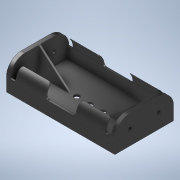
# Autodesk Inventor part: Main body
Saved by Autodesk Inventor 2020 (Build 240168000, 168)
## iProperties
Created: 2021-12-31
Part Number: Main body
Material: ABS Plastic
Document SubType Name: Modeling
Designer: robur
Density: 1.06 g/cm^3
Appearance: Asphalt 2
Author: robur
Autodesk Inventor part; units mm, degrees
ref_plane "YZ Plane" through (0, 0, 0) normal (1, 0, 0) x (0, 1, 0)
sketch "Sketch2" plane through (0, 0, 0) normal (0, 1, 0) x (-1, 0, 0)
  line L0 (28.8, 15.6) -> (-28.8, 15.6)
  line L1 (-28.8, 15.6) -> (-28.8, -15.6)
  line L2 (-28.8, -15.6) -> (28.8, -15.6)
  line L3 (28.8, -15.6) -> (28.8, 15.6)
  line L4 (28.8, 15.6) -> (-28.8, -15.6) construction
  line L5 (-28.8, 15.6) -> (28.8, -15.6) construction
  circle A0 centre (7, 0) radius 1.4
  circle A1 centre (0, 0) radius 1.4
  circle A2 centre (-7, 0) radius 1.4
  dimension "d0" = 57.6
  dimension "d1" = 31.2
  dimension "d2" = 2.8
  dimension "d3" = 21.8
  dimension "d4" = 2.8
  dimension "d5" = 2.8
  dimension "d6" = 7
  dimension "d7" = 7
  constraints: 12 end point, 3 centre point, 2 midpoint, 2 parallel, 1 coincident, 1 horizontal, 1 perpendicular
  measures "d0" distance of L2.end L1.end
  measures "d1" distance of L1.end L0.end
  measures "d2" diameter of A0
  measures "d3" distance from line of A0.centre L3
  measures "d4" diameter of A1
  measures "d5" diameter of A2
  measures "d6" distance of A2.centre point (0, 0)
  measures "d7" distance of point (0, 0) A0.centre
extrude "Extrusion1" add sketch "Sketch2" along normal blind 15
fillet "Fillet1" radius 8 2 edges at (0, 15, 15.6) (0, 15, -15.6)
ref_plane "Work Plane1" through (26.8, 0, 15.6) normal (1, 0, 0) x (0, 0, -1)
sketch "Sketch3" plane through (26.8, 0, 15.6) normal (1, 0, 0) x (0, 0, -1)
  arc A0 (8, 15) -> (0, 7) centre (8, 7) ccw
  arc A1 (8, 15) -> (0, 7) centre (8, 7) ccw projected
  arc A2 (8, 14) -> (1, 7) centre (8, 7) ccw
  arc A3 (31.2, 7) -> (23.2, 15) centre (23.2, 7) ccw projected
  arc A4 (30.2, 7) -> (23.2, 14) centre (23.2, 7) ccw
  line L0 (1, 7) -> (1, 1)
  line L1 (31.2, 0) -> (0, 0) projected
  line L2 (1, 1) -> (30.2, 1)
  line L3 (31.2, 0) -> (31.2, 7) projected
  line L4 (30.2, 1) -> (30.2, 7)
  line L5 (23.2, 15) -> (8, 15)
  line L6 (23.2, 14) -> (8, 14)
  point P0 (15.6, 0)
  dimension "d12" = 7
  dimension "d13" = 7
  dimension "d14" = 6
  dimension "d15" = 29.2
  constraints: 10 end point, 6 point on circle, 3 centre point, 3 coincident, 2 perpendicular, 1 horizontal, 1 parallel, 1 tangent
  measures "d12" radius of A2
  measures "d13" radius of A4
  measures "d14" distance of L0.start L0.end
  measures "d15" distance of L0.end L2.end
extrude "Extrusion2" cut sketch "Sketch3" against normal blind 53.6
sketch "Sketch4" plane through (0, 15, 0) normal (0, 1, 0) x (1, 0, 0)
  line L0 (26.8, -14.6) -> (26.8, 14.6) projected
  line L1 (-26.8, -12.5) -> (26.8, -12.5)
  line L2 (26.8, -12.5) -> (26.8, 12.5)
  line L3 (26.8, 12.5) -> (-26.8, 12.5)
  line L4 (-26.8, 12.5) -> (-26.8, -12.5)
  line L5 (-26.8, -12.5) -> (26.8, 12.5) construction
  line L6 (26.8, -12.5) -> (-26.8, 12.5) construction
  point P0 (0, 0)
  dimension "d51" = 25
  constraints: 12 end point, 2 midpoint, 2 parallel, 1 horizontal, 1 perpendicular, 1 point on line
  measures "d51" distance of L3.end L1.start
extrude "Extrusion3" cut sketch "Sketch4" against normal blind 3
ref_plane "Work Plane2" through (28.8, 0, -15.6) normal (0, 0, -1) x (-1, 0, 0)
sketch "Sketch8" plane through (-26.8, 0, 15.6) normal (1, 0, 0) x (0, 0, -1)
  line L0 (3.1, 13.3238) -> (3.1, 12) projected
  arc A0 (3.1, 13.0156) -> (1, 7) centre (6.8512, 8.3318) ccw
  line L1 (8, 15) -> (23.2, 15) projected
  line L2 (15.6, 15) -> (15.6, 0.9201)
  arc A1 (30.2, 7) -> (28.1, 13.0156) centre (24.3488, 8.3318) ccw
  line L3 (28.1, 13.0156) -> (3.1, 13.0156)
  arc A2 (30.2, 7) -> (28.099, 12) centre (23.2, 7) ccw projected
  line L4 (1, 7) -> (30.2, 7)
  point P0 (15.6, 0)
  constraints: 6 end point, 4 point on circle, 3 symmetric about line, 2 centre point, 1 horizontal, 1 midpoint, 1 parallel, 1 point on line, 1 vertical, 1 other
extrude "Extrusion6" cut sketch "Sketch8" along normal blind 53.6
sketch "Sketch9" plane through (28.8, 0, -15.6) normal (0, 0, -1) x (-1, 0, 0)
  line L0 (2, 13.3238) -> (5, 13.3238)
  line L1 (5, 11.8238) -> (5, 8.2996)
  line L2 (3.5, 6.7996) -> (2, 6.7996)
  line L3 (2, 6.7996) -> (2, 13.3238)
  arc A0 (3.5, 6.7996) -> (5, 8.2996) centre (3.5, 8.2996) ccw
  arc A1 (6.5, 13.3238) -> (5, 11.8238) centre (6.5, 11.8238) ccw
  line L4 (5, 13.3238) -> (6.5, 13.3238)
  line L5 (28.8, 0) -> (28.8, 13.3238)
  line L6 (55.6, 13.3238) -> (52.6, 13.3238)
  line L7 (52.6, 11.8238) -> (52.6, 8.2996)
  line L8 (54.1, 6.7996) -> (55.6, 6.7996)
  line L9 (55.6, 6.7996) -> (55.6, 13.3238)
  arc A2 (52.6, 8.2996) -> (54.1, 6.7996) centre (54.1, 8.2996) ccw
  arc A3 (52.6, 11.8238) -> (51.1, 13.3238) centre (51.1, 11.8238) ccw
  line L10 (52.6, 13.3238) -> (51.1, 13.3238)
  line L11 (55.6, 13.3238) -> (2, 13.3238) projected
  line L12 (2, 7) -> (55.6, 7) projected
  line L13 (20.85, 13.3238) -> (36.75, 13.3238)
  line L14 (36.75, 11.8238) -> (36.75, 8.5)
  line L15 (35.25, 7) -> (22.35, 7)
  line L16 (20.85, 8.5) -> (20.85, 11.8238)
  arc A4 (20.85, 8.5) -> (22.35, 7) centre (22.35, 8.5) ccw
  arc A5 (35.25, 7) -> (36.75, 8.5) centre (35.25, 8.5) ccw
  arc A6 (38.25, 13.3238) -> (36.75, 11.8238) centre (38.25, 11.8238) ccw
  arc A7 (20.85, 11.8238) -> (19.35, 13.3238) centre (19.35, 11.8238) ccw
  line L17 (20.85, 13.3238) -> (19.35, 13.3238)
  line L18 (36.75, 13.3238) -> (38.25, 13.3238)
  point P0 (53.3509, 7)
  point P1 (4.2491, 7)
  dimension "d55" = 3
  dimension "d57" = 1.5
  dimension "d58" = 1.5
  dimension "d59" = 3
  dimension "d60" = 1.5
  dimension "d63" = 15.85
  dimension "d64" = 3
  dimension "d65" = 1.5
  dimension "d66" = 1.5
  dimension "d67" = 3
  dimension "d68" = 1.5
  dimension "d69" = 1.5
  dimension "d70" = 3
  dimension "d71" = 1.5
  dimension "d72" = 1.5
  dimension "d73" = 3
  dimension "d74" = 1.5
  dimension "d75" = 1.5
  constraints: 34 end point, 16 point on circle, 9 symmetric about line, 8 centre point, 4 parallel, 2 horizontal, 2 perpendicular, 6 other
  measures "d55" diameter of A0
  measures "d57" distance from line of L1 A0.centre
  measures "d58" distance from line of L2 A0.centre
  measures "d59" diameter of A1
  measures "d60" distance from line of L1 A1.centre
  measures "d63" distance between parallel lines of L7 L14
  measures "d64" diameter of A4
  measures "d65" distance from line of L12 A4.centre
  measures "d66" distance from line of L16 A4.centre
  measures "d67" diameter of A5
  measures "d68" distance from line of L14 A5.centre
  measures "d69" distance from line of L12 A5.centre
  measures "d70" diameter of A6
  measures "d71" distance from line of L14 A6.centre
  measures "d72" distance from line of L13 A6.centre
  measures "d73" diameter of A7
  measures "d74" distance from line of L16 A7.centre
  measures "d75" distance from line of L13 A7.centre
extrude "Extrusion7" cut sketch "Sketch9" against normal blind 53.8 contours L0 L4 A1 L1 A0 L12 L3 | L11 L5 L12 A4 L16 A7 | L5 L11 A6 L14 A5 L12 | A2 L7 A3 L10 L6 L9 L12
sketch "Sketch10" plane through (26.8, 1, 14.6) normal (0, 1, 0) x (1, 0, 0)
  line L0 (0, 0) -> (0, 29.2) projected
  line L1 (0, 14.1) -> (0, 15.1)
  line L2 (-53.6, 15.1) -> (-53.6, 14.1)
  circle A0 centre (-26.8, 14.6) radius 1.4 projected
  line L3 (-53.6, 14.1) -> (0, 15.1) construction
  line L4 (0, 14.1) -> (-53.6, 15.1) construction
  line L5 (-37.3, 14.1) -> (-37.3, 15.1)
  circle A1 centre (-33.8, 14.6) radius 1.4 projected
  line L6 (-16.3, 15.1) -> (-16.3, 14.1)
  circle A2 centre (-19.8, 14.6) radius 1.4 projected
  line L7 (-53.6, 14.1) -> (-37.3, 14.1)
  line L8 (-16.3, 14.1) -> (0, 14.1)
  line L9 (0, 15.1) -> (-16.3, 15.1)
  line L10 (-37.3, 15.1) -> (-53.6, 15.1)
  dimension "d78" = 1
  dimension "d79" = 3.5
  dimension "d80" = 3.5
  constraints: 20 end point, 6 perpendicular, 5 parallel, 2 horizontal, 2 midpoint, 1 point on line
  measures "d78" distance of L1.end L1.start
  measures "d79" distance from line of L5 A1.centre
  measures "d80" distance from line of L6 A2.centre
extrude "Extrusion8" add sketch "Sketch10" along normal blind 14 contours L8 L6 L9 L0 | L10 L5 L7 L2
sketch "Sketch11" plane through (-26.8, 1, 0.5) normal (0, 0, 1) x (1, 0, 0)
  line L0 (16.3, 14) -> (0, 14) projected
  line L1 (16.3, 0) -> (0, 0) projected
  line L2 (0, 14) -> (16.3, 0)
  line L3 (16.3, 0) -> (16.3, 14)
  line L4 (20.35, 6) -> (2.2491, 6) projected
  line L5 (0, 14) -> (16.3, 14) projected
  line L6 (16.3, 14) -> (0, 14)
  point P0 (26.8, -1)
  constraints: 6 end point, 2 perpendicular
extrude "Extrusion9" cut sketch "Sketch11" against normal blind 1
sketch "Sketch12" plane through (10.5, 1, 0.5) normal (0, 0, 1) x (1, 0, 0)
  line L0 (16.3, 0) -> (0, 0) projected
  line L1 (16.3, 14) -> (0, 0)
  line L2 (0, 14) -> (16.3, 14) projected
  line L3 (0, 0) -> (0, 14)
  line L4 (16.3, 0) -> (16.3, 14) projected
  line L5 (0, 14) -> (16.3, 14)
  point P0 (-10.5, -1)
  constraints: 6 end point, 2 perpendicular
extrude "Extrusion10" cut sketch "Sketch12" against normal blind 1 contours L3 L2 L1
sketch "Sketch13" plane through (28.8, 0, 15.6) normal (1, 0, 0) x (0, 0, -1)
  circle A0 centre (8, 7.8) radius 0.9
  line L0 (8, 15) -> (23.2, 15) projected
  line L1 (0, 0) -> (0, 7) projected
  line L2 (15.6, 0) -> (15.6, 15)
  line L3 (31.2, 0) -> (31.2, 7) projected
  circle A1 centre (23.2, 7.8) radius 0.9
  dimension "d87" = 1.8
  dimension "d88" = 7.2
  dimension "d89" = 8
  dimension "d90" = 15.6
  dimension "d91" = 15.6
  constraints: 2 centre point, 2 end point, 1 midpoint, 1 symmetric about line, 1 other
  measures "d87" diameter of A0
  measures "d88" distance from line of L0 A0.centre
  measures "d89" distance from line of L1 A0.centre
  measures "d90" distance between parallel lines of L2 L1
  measures "d91" distance between parallel lines of L3 L2
extrude "Extrusion11" cut sketch "Sketch13" against normal blind 2
sketch "Sketch14" plane through (-26.8, 0, 15.6) normal (1, 0, 0) x (0, 0, -1)
  circle A0 centre (8, 7.8) radius 0.9 projected
  circle A1 centre (8, 7.8) radius 0.9
  circle A2 centre (23.2, 7.8) radius 0.9 projected
  circle A3 centre (23.2, 7.8) radius 0.9
  point P0 (15.6, 0)
  constraints: 2 centre point, 2 coincident
extrude "Extrusion12" cut sketch "Sketch14" against normal blind 2
body "Solid1"
